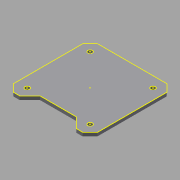
# Autodesk Inventor part: compactActiveLoad_BottomCover
Saved by Autodesk Inventor 2013 (Build 170138000, 138)
## iProperties
Created: 2015-06-14
Part Number: compactActiveLoad_BottomCover
Material: Generic
Document SubType Name: Modeling
Designer: Masta
Density: 1 g/cm^3
Author: Masta
Autodesk Inventor part; units mm, degrees
ref_plane "YZ Plane" through (0, 0, 0) normal (1, 0, 0) x (0, 1, 0)
ref_plane "XZ Plane" through (0, 0, 0) normal (0, 1, 0) x (-1, 0, 0)
ref_plane "XY Plane" through (0, 0, 0) normal (0, 0, 1) x (1, 0, 0)
sketch "Sketch1" plane through (0, 0, 0) normal (0, 0, 1) x (1, 0, 0)
  line L0 (29, 29) -> (-29, 29)
  line L1 (-29, 29) -> (-29, -29)
  line L2 (-29, -29) -> (29, -29)
  line L3 (29, -29) -> (29, 29)
  line L4 (29, 29) -> (-29, -29) construction
  line L5 (-29, 29) -> (29, -29) construction
  line L6 (21.7, -21.7) -> (-21.7, -21.7) construction
  line L7 (-21.7, -21.7) -> (-21.7, 21.7) construction
  line L8 (-21.7, 21.7) -> (21.7, 21.7) construction
  line L9 (21.7, 21.7) -> (21.7, -21.7) construction
  line L10 (21.7, -21.7) -> (-21.7, 21.7) construction
  line L11 (-21.7, -21.7) -> (21.7, 21.7) construction
  line L12 (-12.5, -36) -> (12.5, -36)
  line L13 (12.5, -36) -> (12.5, -22)
  line L14 (12.5, -22) -> (-12.5, -22)
  line L15 (-12.5, -22) -> (-12.5, -36)
  line L16 (-12.5, -36) -> (12.5, -22) construction
  line L17 (12.5, -36) -> (-12.5, -22) construction
  point P0 (0, 0)
  point P1 (0, -29)
  dimension "d0" = 58
  dimension "d1" = 58
  dimension "d7" = 43.4
  dimension "d15" = 25
  dimension "d16" = 14
  constraints: 36 end point, 7 midpoint, 6 parallel, 4 coincident, 4 perpendicular, 3 horizontal
  measures "d0" distance of L2.end L1.end
  measures "d1" distance of L1.end L0.end
  measures "d7" distance of L7.end L8.end
  measures "d15" distance of L14.end L13.end
  measures "d16" distance of L13.end L12.end
extrude "Extrusion1" add sketch "Sketch1" along normal blind 2.55 contours L3 L2 L13 L14 L15 L1 L0 | L2 L15 L14 L13
chamfer "Chamfer1" distance 5 angle 45 4 edges at (29, 29, 1.275) (-29, 29, 1.275) (-29, -29, 1.275) (29, -29, 1.275)
hole "Hole1" at (-21.7, 21.7, 0) at (-21.7, -21.7, 0) at (21.7, -21.7, 0) at (21.7, 21.7, 0) direction (0, 0, 1) diameter 3.2 end through all
extrude "Extrusion2" cut sketch "Sketch1" along normal up to next contours L13 L12 L15 L2 | L2 L15 L14 L13
chamfer "Chamfer2" distance 7 angle 45 2 edges at (-12.5, -29, 1.275) (12.5, -29, 1.275)
sketch "Sketch2" plane through (0, 0, 2.55) normal (0, 0, 1) x (1, 0, 0)
  line L0 (19.5, -29) -> (12.5, -22) projected
  line L1 (19.5, -29) -> (24, -29) projected
  line L2 (29, -24) -> (24, -29) projected
  line L3 (29, -24) -> (29, 24) projected
  line L4 (24, 29) -> (29, 24) projected
  line L5 (24, 29) -> (-24, 29) projected
  line L6 (-29, 24) -> (-24, 29) projected
  line L7 (-29, 24) -> (-29, -24) projected
  line L8 (-24, -29) -> (-29, -24) projected
  line L9 (-24, -29) -> (-19.5, -29) projected
  line L10 (-12.5, -22) -> (-19.5, -29) projected
  line L11 (-12.5, -22) -> (12.5, -22) projected
  circle A0 centre (21.7, 21.7) radius 1.6 projected
  circle A1 centre (-21.7, -21.7) radius 1.6 projected
  circle A2 centre (-21.7, 21.7) radius 1.6 projected
  circle A3 centre (21.7, -21.7) radius 1.6 projected
  point P0 (0, 0)
body "Solid1"
